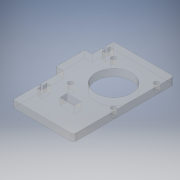
# Autodesk Inventor part: Belt_Holder2
Saved by Autodesk Inventor 2016 (Build 200138000, 138)
## iProperties
Created: 2018-05-31
Part Number: Belt_Holder2
Material: Polycarbonate, Clear
Document SubType Name: Modeling
Designer: Phil Erle
Density: 1.2 g/cm^3
Appearance: Polycarbonate - Clear
Author: Phil Erle
Autodesk Inventor part; units mm, degrees
ref_plane "YZ Plane" through (0, 0, 0) normal (1, 0, 0) x (0, 1, 0)
ref_plane "XZ Plane" through (0, 0, 0) normal (0, 1, 0) x (-1, 0, 0)
ref_plane "XY Plane" through (0, 0, 0) normal (0, 0, 1) x (1, 0, 0)
sketch "Sketch1" plane through (0, 0, 0) normal (0, 0, 1) x (1, 0, 0)
  line L0 (20, 35) -> (-20, 35)
  line L1 (-20, 35) -> (-20, 20)
  line L2 (-20, 20) -> (-25, 20)
  line L3 (-25, 20) -> (-25, 0)
  line L4 (-25, 0) -> (-20, 0)
  line L5 (-20, 0) -> (-20, -35)
  line L6 (-20, -35) -> (20, -35)
  line L7 (22, -33) -> (22, 33)
  arc A0 (22, 33) -> (20, 35) centre (20, 33) ccw
  arc A1 (20, -35) -> (22, -33) centre (20, -33) ccw
  point P0 (0, 0)
  point P1 (22, 35)
  point P2 (22, -35)
  point P3 (22, 0)
  point P4 (0, 35)
  dimension "d0" = 70
  dimension "d1" = 5
  dimension "d2" = 20
  dimension "d3" = 15
  dimension "d4" = 42
  dimension "d7" = 2
  constraints: 16 end point, 6 perpendicular, 6 point on line, 4 point on circle, 4 tangent, 2 centre point, 2 midpoint, 1 equal radius, 1 horizontal, 1 horizontal alignment, 1 vertical alignment
  measures "d0" distance of point (22, -35) point (22, 35)
  measures "d1" distance between parallel lines of L3 L1
  measures "d2" distance of L2.end L3.end
  measures "d3" distance between parallel lines of L0 L2
  measures "d4" distance of point (22, 35) L0.end
  measures "d7" radius of A0
extrude "Extrusion1" add sketch "Sketch1" along normal blind 5
sketch "Sketch2" plane through (0, 0, 5) normal (0, 0, 1) x (1, 0, 0)
  point P0 (0, 0)
  point P1 (5, 10)
  dimension "d8" = 10
  dimension "d9" = 5
  measures "d8" vertical distance of point (5, 10) point (0, 0)
  measures "d9" horizontal distance of point (0, 0) point (5, 10)
hole "Hole1" at (5, 10, 5) direction (0, 0, -1) diameter 25 depth 8 tip angle 118
sketch "Sketch3" plane through (0, 0, 5) normal (0, 0, 1) x (1, 0, 0)
  circle A0 centre (5, 10) radius 12.5 projected
  line L0 (-10, -5) -> (20, -5) construction
  line L1 (20, -5) -> (20, 25) construction
  line L2 (20, 25) -> (-10, 25) construction
  line L3 (-10, 25) -> (-10, -5) construction
  line L4 (-10, -5) -> (20, 25) construction
  line L5 (20, -5) -> (-10, 25) construction
  point P0 (0, 0)
  dimension "d17" = 30
  dimension "d18" = 30
  constraints: 12 end point, 4 coincident, 2 midpoint, 2 parallel, 1 horizontal, 1 perpendicular
  measures "d17" distance of L1.end L2.end
  measures "d18" distance of L0.end L1.end
hole "Hole2" at (-10, 25, 5) at (20, 25, 5) at (20, -5, 5) at (-10, -5, 5) direction (0, 0, -1) diameter 3.4 depth 8 tip angle 118 clearance for "Countersunk Flat Head Screw DIN EN ISO 2009" size "M3" standard "DIN"
sketch "Sketch4" plane through (0, 0, 5) normal (0, 0, 1) x (1, 0, 0)
  line L0 (-20, 20) -> (-20, 35) projected
  line L1 (-20, 29.0072) -> (-18.2028, 29.0072)
  line L2 (-18.2028, 29.0072) -> (-18.2028, 30.672)
  line L3 (-18.2028, 30.672) -> (-15.6132, 30.672)
  line L4 (-15.6132, 30.672) -> (-15.6132, 25.2153)
  line L5 (-15.6132, 25.2153) -> (-18.2028, 25.2153)
  line L6 (-18.2028, 25.2153) -> (-18.2028, 26.88)
  line L7 (-18.2028, 26.88) -> (-20, 26.88)
  line L8 (-20, 26.88) -> (-20, 29.0072)
  line L9 (-20, -35) -> (-20, 0) projected
  line L10 (-20, -15.9413) -> (-18.2028, -15.9413)
  line L11 (-18.2028, -15.9413) -> (-18.2028, -13.3517)
  line L12 (-18.2028, -13.3517) -> (-15.6132, -13.3517)
  line L13 (-15.6132, -13.3517) -> (-15.6132, -19.7333)
  line L14 (-15.6132, -19.7333) -> (-18.2028, -19.7333)
  line L15 (-18.2028, -19.7333) -> (-18.2028, -17.5)
  line L16 (-18.2028, -17.5) -> (-20, -17.5)
  line L17 (-20, -17.5) -> (-20, -15.9413)
  point P0 (0, 0)
  constraints: 32 end point, 9 perpendicular, 5 point on line, 3 horizontal, 2 collinear, 1 midpoint
extrude "Extrusion2" cut sketch "Sketch4" against normal blind 5
sketch "Sketch5" plane through (0, 0, 5) normal (0, 0, 1) x (1, 0, 0)
  line L0 (-5, -17.5) -> (5, -17.5)
  line L1 (5, -17.5) -> (5, -12.5)
  line L2 (5, -12.5) -> (-5, -12.5)
  line L3 (-5, -12.5) -> (-5, -17.5)
  line L4 (-5, -17.5) -> (5, -12.5) construction
  line L5 (5, -17.5) -> (-5, -12.5) construction
  point P0 (0, 0)
  point P1 (0, -15)
  point P2 (0, -15)
  dimension "d28" = 10
  dimension "d29" = 5
  dimension "d30" = 15
  constraints: 12 end point, 3 midpoint, 2 parallel, 1 horizontal, 1 perpendicular, 1 vertical alignment
  measures "d28" distance of L2.end L1.end
  measures "d29" distance of L1.end L0.end
  measures "d30" distance of point (0, 0) point (0, -15)
extrude "Extrusion3" cut sketch "Sketch5" against normal blind 5
body "Solid1"
